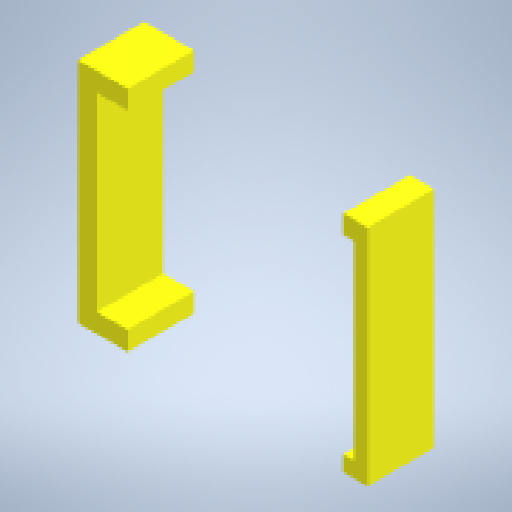
# Autodesk Inventor part: pitop hold
Saved by Autodesk Inventor 2024 (Build 280153000, 153)
## iProperties
Created: 2024-01-06
Part Number: pitop hold
Material: Generic
Document SubType Name: Modeling
Designer: student
Density: 1 g/cm^3
Appearance: Yellow
Author: student
Autodesk Inventor part; units mm, degrees
ref_plane "YZ Plane" through (0, 0, 0) normal (1, 0, 0) x (0, 1, 0)
ref_plane "XZ Plane" through (0, 0, 0) normal (0, 1, 0) x (-1, 0, 0)
ref_plane "XY Plane" through (0, 0, 0) normal (0, 0, 1) x (1, 0, 0)
sketch "Sketch1" plane through (0, 0, 0) normal (0, 0, 1) x (1, 0, 0)
  line L0 (-53.1764, 61.1751) -> (-53.1764, 48.4751) projected
  line L1 (-53.1764, 48.4751) -> (83.9836, 48.4751) projected
  line L2 (-53.1764, 150.0751) -> (-53.1764, 137.3751) projected
  line L3 (83.9836, 150.0751) -> (-53.1764, 150.0751) projected
  line L4 (-53.1764, 61.1751) -> (-53.1764, 48.4751)
  line L5 (-53.1764, 61.1751) -> (-53.1764, 79.1879)
  line L6 (-36.6444, 48.4751) -> (-36.6444, 38.302)
  line L7 (-36.6444, 38.302) -> (-63.3364, 38.302)
  line L8 (-63.3364, 38.302) -> (-63.3364, 79.1879)
  line L9 (83.9836, 150.0751) -> (83.9836, 48.4751)
  line L10 (78.719, 48.4751) -> (78.719, 40.2129)
  line L11 (78.719, 40.2129) -> (91.6764, 40.2129)
  line L12 (91.6764, 40.2129) -> (91.6764, 160.0146)
  line L13 (91.6764, 160.0146) -> (78.719, 160.0146)
  line L14 (78.719, 160.0146) -> (78.719, 150.0751)
  line L15 (83.9836, 150.0751) -> (78.719, 150.0751)
  line L16 (-53.1764, 79.1879) -> (-53.1764, 150.0751)
  line L17 (-36.6444, 150.0751) -> (-36.6444, 160.0146)
  line L18 (-36.6444, 160.0146) -> (-63.3364, 160.0146)
  line L19 (-63.3364, 160.0146) -> (-63.3364, 79.1879)
  point P0 (0, 0)
  dimension "d0" = 10.16
  constraints: 32 end point, 7 perpendicular, 7 point on line, 4 vertical, 2 collinear, 1 parallel
  measures "d0" distance of L5.end L8.end
extrude "Extrusion1" add sketch "Sketch1" along normal blind 35.56 contours L0 L1 L6 L7 L8 L19 L18 L17 L3 L2 L16 L5 | L1 L9 L3 L14 L13 L12 L11 L10
body "Solid1"
